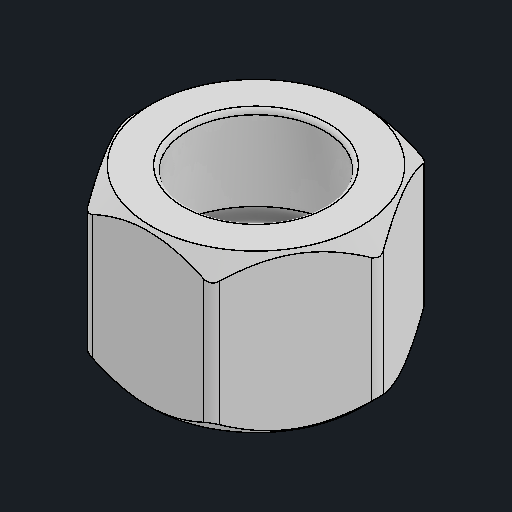
# Autodesk Inventor part: 40mm Nut
Saved by Autodesk Inventor 2026.2 (Build 302298000, 298)
## iProperties
Created: 2026-06-22
Part Number: 40mm Nut
Material: Generic
Document SubType Name: Modeling
Designer: Joshua Eah
Density: 1 g/cm^3
Appearance: Default
Author: Joshua Eah
Autodesk Inventor part; units mm, degrees
ref_plane "YZ Plane" through (0, 0, 0) normal (1, 0, 0) x (0, 1, 0)
ref_plane "XZ Plane" through (0, 0, 0) normal (0, 1, 0) x (-1, 0, 0)
sketch "Sketch1" plane through (0, 0, 0) normal (0, 1, 0) x (-1, 0, 0)
  circle A0 centre (0, 0) radius 22.5
  circle A1 centre (0, 0) radius 27.5
  line L0 (-15.8771, -27.5) -> (-31.7543, 0)
  line L1 (-31.7543, 0) -> (-15.8771, 27.5)
  line L2 (-15.8771, 27.5) -> (15.8771, 27.5)
  line L3 (15.8771, 27.5) -> (31.7543, 0)
  line L4 (31.7543, 0) -> (15.8771, -27.5)
  line L5 (15.8771, -27.5) -> (-15.8771, -27.5)
  point P0 (0, -27.5)
  point P1 (23.8157, -13.75)
  point P2 (-23.8157, -13.75)
  point P3 (23.8157, 13.75)
  point P4 (0, 27.5)
  point P5 (-23.8157, 13.75)
  dimension "d0" = 45
  dimension "d1" = 55
  constraints: 12 end point, 2 centre point, 2 coincident, 1 concentric, 1 horizontal, 1 tangent, 13 other
  measures "d0" diameter of A0
  measures "d1" diameter of A1
extrude "Extrusion1" add sketch "Sketch1" against normal blind 15
extrude "Extrusion2" add sketch "Sketch1" along normal blind 25 separate body
draft "FaceDraft1" angle 12 pull direction (0, -1, 0) faces at (-22.2086, 16.6667, -3.6093) fixed edges at (22.5, 0, 0) (22.5, 0, 0)
combine bodies "Combine1" operation type add bodies to combine 1 2
ref_plane "Work Plane2" through (-15.8771, -15, 0) normal (0, 0, 1) x (1, 0, 0)
sketch "Sketch2" plane through (-15.8771, -15, 0) normal (0, 0, 1) x (1, 0, 0)
  line L0 (31.7543, 0) -> (31.7543, 40) projected
  line L1 (47.6314, 0) -> (31.7543, 0) projected
  line L2 (47.6314, 40) -> (47.6314, 0) projected
  line L3 (31.7543, 40) -> (47.6314, 40) projected
  line L4 (42.6314, 40) -> (47.6314, 35)
  line L5 (47.6314, 20) -> (31.7543, 20)
  line L6 (42.6314, 0) -> (47.6314, 5)
  line L7 (15.8771, -8) -> (15.8771, 48) projected
  point P0 (47.6314, 5)
  point P1 (42.6314, 0)
  dimension "d11" = 45
  dimension "d12" = 5
  constraints: 6 end point, 2 midpoint, 2 point on line, 2 symmetric about line
  measures "d11" angle of L3 L4
  measures "d12" distance from line of L2 L4.start
revolve "Revolution1" cut sketch "Sketch2" angle 360 about axis through (0, -10, 0) along (0, 1, 0) bodies 1 contours L6 L2 L1 | L3 L2 L4
fillet "Fillet2" radius 3 6 edges at (15.8771, 5, -27.5) (31.7543, 5, 0) (-15.8771, 5, -27.5) (-31.7543, 5, 0) (15.8771, 5, 27.5) (-15.8771, 5, 27.5)
fillet "Fillet2" radius 1 2 edges at (22.5, -15, 0) (17.1861, 25, 0)
thread "Thread2" size "M45x4.5" class "6H" standard "ANSI Metric M Profile" length 15
body "Solid1"
